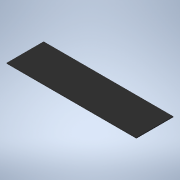
# Autodesk Inventor part: FGR AL-2-PGN-plus-P 160 WKST,PGN-plus-P 160-2-AS-P18Aluminium6.5110452001216049.51650000000000000000
Saved by Autodesk Inventor 2021 (Build 250183000, 183)
## iProperties
Created: 2025-07-30
Part Number: FGR AL-2-PGN-plus-P 160 WKST,PGN-plus-P 160-2-AS-P18Aluminium6.5110452001216049.51650000000000000000
Material: Generic
Catalog Web Link: www.cadenas.de
Description: FGR-Customizable gripper fingers
Vendor: SCHUNK
Document SubType Name: Modeling
Designer: psAdmin
Manufacturer: SCHUNK
Mass: 7.755 g
Surface Area: 159.34 cm^2
Volume: 7.755 cm^3
Density: 1 g/cm^3
Appearance: PSOLRGB-175-175-175
Category: PARTsolutions
Company: SCHUNK
Title: FGR AL-2-PGN-plus-P 160, 110452002
Author: Cadenas PARTsolutions
Comments: Customizable gripper fingers
PSOL_IDENT_0: {$CADENAS_DATA/23d-libs/schunk/greifsysteme/konfigurationen/system_baukasten/easy_finger/easy_finger
PSOL_IDENT_1: _ring.prj},476 {VTYP=3D},{NB=FGR AL-2-PGN-plus-P 160 WKST,PGN-plus-P 160-2-AS-P18Aluminium6.51104520
PSOL_IDENT_2: 01216049.51650000000000000000},{LINA=FGR AL-2-PGN-plus-P 160, 110452002},{NN=FGR},{DATE=13.11.2024 0
PSOL_IDENT_3: 9:26:27},{GEOMDATE=20.06.2024 14:58:27},{VERSION=},{LINEID=10},{WBVAR=BR,BGVR,ASIS,SPANNKONT,CNSMAT,
PSOL_IDENT_4: HUB,RH,X,Y,Z,ABK,DWS,GFL,GFT,PP,PW,RA,EFO,FASE1,FL1,FASE2,FL2,FASE3,FW3,FL3,FASE4,FW4,FL4,WAERMEBE,B
PSOL_IDENT_5: M},{WBNUMERIC=HUB,RH,X,Y,Z,ABK,DWS,GFL,GFT,PP,PW,RA,EFO,FL1,FL2,FASE3,FW3,FL3,FW4,FL4,BM}  {NB=FGR A
PSOL_IDENT_6: L-2-PGN-plus-P 160 WKST,PGN-plus-P 160-2-AS-P18Aluminium6.5110452001216049.51650000000000000000},{LI
PSOL_IDENT_7: NA=FGR AL-2-PGN-plus-P 160, 110452002},{KT=DUMMY},{START=Geometriemodell 2},{VERSION=1},{VER=V1},{MA
PSOL_IDENT_8: TN=3786171200_fgr_gl_ia_v1},{XMLMATN=material|},{XMLMAT=AlZn55MgCu_EN-AW-7075_34365},{TYP=FGR AL-2-P
PSOL_IDENT_9: GN-plus-P 160},{TYPX=PGN-plus-P 160},{TYPXX=PGN-plus-P 160},{TYPXMAT=AL},{BR=PGN-plus-P},{BG=160.0},
PSOL_IDENT_10: {BGVR=PGN-plus-P 160-2-AS-P},{BGVRX='PGN-plus-P 40','PGN-plus-P 40','PGN-plus-P 40-SD','PGN-plus-P 4
PSOL_IDENT_11: 0-SD','PGN-plus-P 40-K','PGN-plus-P 40-K','PGN-plus-P 40-V','PGN-plus-P 40-V','PGN-plus-P 40-P','PGN
PSOL_IDENT_12: -plus-P 40-P','PGN-plus-P 40-AS','PGN-plus-P 40-AS','PGN-plus-P 40-AS-SD','PGN-plus-P 40-AS-SD','PGN
PSOL_IDENT_13: -plus-P 40-AS-K','PGN-plus-P 40-AS-K','PGN-plus-P 40-AS-V','PGN-plus-P 40-AS-V','PGN-plus-P 40-AS-P'
PSOL_IDENT_14: ,'PGN-plus-P 40-AS-P','PGN-plus-P 40-IS','PGN-plus-P 40-IS','PGN-plus-P 40-IS-SD','PGN-plus-P 40-IS-
PSOL_IDENT_15: SD','PGN-plus-P 40-IS-K','PGN-plus-P 40-IS-K','PGN-plus-P 40-IS-V','PGN-plus-P 40-IS-V','PGN-plus-P
PSOL_IDENT_16: 50-1','PGN-plus-P 50-1','PGN-plus-P 50-1-SD','PGN-plus-P 50-1-SD','PGN-plus-P 50-1-K','PGN-plus-P 50
PSOL_IDENT_17: -1-K','PGN-plus-P 50-1-V','PGN-plus-P 50-1-V','PGN-plus-P 50-1-P','PGN-plus-P 50-1-P','PGN-plus-P 50
PSOL_IDENT_18: -2','PGN-plus-P 50-2','PGN-plus-P 50-2-SD','PGN-plus-P 50-2-SD','PGN-plus-P 50-2-K','PGN-plus-P 50-2
PSOL_IDENT_19: -K','PGN-plus-P 50-2-V','PGN-plus-P 50-2-V','PGN-plus-P 50-2-P','PGN-plus-P 50-2-P','PGN-plus-P 50-1
PSOL_IDENT_20: -AS','PGN-plus-P 50-1-AS','PGN-plus-P 50-1-AS-SD','PGN-plus-P 50-1-AS-SD','PGN-plus-P 50-1-AS-K','PG
PSOL_IDENT_21: N-plus-P 50-1-AS-K','PGN-plus-P 50-1-AS-V','PGN-plus-P 50-1-AS-V','PGN-plus-P 50-1-AS-P','PGN-plus-P
PSOL_IDENT_22: 50-1-AS-P','PGN-plus-P 50-2-AS','PGN-plus-P 50-2-AS','PGN-plus-P 50-2-AS-SD','PGN-plus-P 50-2-AS-SD'
PSOL_IDENT_23: ,'PGN-plus-P 50-2-AS-K','PGN-plus-P 50-2-AS-K','PGN-plus-P 50-2-AS-V','PGN-plus-P 50-2-AS-V','PGN-pl
PSOL_IDENT_24: us-P 50-2-AS-P','PGN-plus-P 50-2-AS-P','PGN-plus-P 50-1-IS','PGN-plus-P 50-1-IS','PGN-plus-P 50-1-IS
PSOL_IDENT_25: -SD','PGN-plus-P 50-1-IS-SD','PGN-plus-P 50-1-IS-K','PGN-plus-P 50-1-IS-K','PGN-plus-P 50-1-IS-V','P
PSOL_IDENT_26: GN-plus-P 50-1-IS-V','PGN-plus-P 50-2-IS','PGN-plus-P 50-2-IS','PGN-plus-P 50-2-IS-SD','PGN-plus-P 5
PSOL_IDENT_27: 0-2-IS-SD','PGN-plus-P 50-2-IS-K','PGN-plus-P 50-2-IS-K','PGN-plus-P 50-2-IS-V','PGN-plus-P 50-2-IS-
PSOL_IDENT_28: V','PGN-plus-P 64-1','PGN-plus-P 64-1','PGN-plus-P 64-1-SD','PGN-plus-P 64-1-SD','PGN-plus-P 64-1-K'
PSOL_IDENT_29: ,'PGN-plus-P 64-1-K','PGN-plus-P 64-1-V','PGN-plus-P 64-1-V','PGN-plus-P 64-1-P','PGN-plus-P 64-1-P'
PSOL_IDENT_30: ,'PGN-plus-P 64-2','PGN-plus-P 64-2','PGN-plus-P 64-2-SD','PGN-plus-P 64-2-SD','PGN-plus-P 64-2-K','
PSOL_IDENT_31: PGN-plus-P 64-2-K','PGN-plus-P 64-2-V','PGN-plus-P 64-2-V','PGN-plus-P 64-2-P','PGN-plus-P 64-2-P','
PSOL_IDENT_32: PGN-plus-P 64-1-AS','PGN-plus-P 64-1-AS','PGN-plus-P 64-1-AS-SD','PGN-plus-P 64-1-AS-SD','PGN-plus-P
PSOL_IDENT_33: 64-1-AS-K','PGN-plus-P 64-1-AS-K','PGN-plus-P 64-1-AS-V','PGN-plus-P 64-1-AS-V','PGN-plus-P 64-1-AS
PSOL_IDENT_34: -P','PGN-plus-P 64-1-AS-P','PGN-plus-P 64-2-AS','PGN-plus-P 64-2-AS','PGN-plus-P 64-1-IS','PGN-plus-
PSOL_IDENT_35: P 64-1-IS','PGN-plus-P 64-1-IS-SD','PGN-plus-P 64-1-IS-SD','PGN-plus-P 64-1-IS-K','PGN-plus-P 64-1-I
PSOL_IDENT_36: S-K','PGN-plus-P 64-1-IS-V','PGN-plus-P 64-1-IS-V','PGN-plus-P 64-2-IS','PGN-plus-P 64-2-IS','PGN-pl
PSOL_IDENT_37: us-P 64-2-IS-SD','PGN-plus-P 64-2-IS-SD','PGN-plus-P 64-2-IS-K','PGN-plus-P 64-2-IS-K','PGN-plus-P 6
PSOL_IDENT_38: 4-2-V','PGN-plus-P 64-2-V','PGN-plus-P 80-1','PGN-plus-P 80-1','PGN-plus-P 80-1-SD','PGN-plus-P 80-1
PSOL_IDENT_39: -SD','PGN-plus-P 80-1-K','PGN-plus-P 80-1-K','PGN-plus-P 80-1-V','PGN-plus-P 80-1-V','PGN-plus-P 80-
PSOL_IDENT_40: 1-P','PGN-plus-P 80-1-P','PGN-plus-P 80-2','PGN-plus-P 80-2','PGN-plus-P 80-2-SD','PGN-plus-P 80-2-S
PSOL_IDENT_41: D','PGN-plus-P 80-2-K','PGN-plus-P 80-2-K','PGN-plus-P 80-2-V','PGN-plus-P 80-2-V','PGN-plus-P 80-2-
PSOL_IDENT_42: P','PGN-plus-P 80-2-P','PGN-plus-P 80-1-AS','PGN-plus-P 80-1-AS','PGN-plus-P 80-1-AS-SD','PGN-plus-P
PSOL_IDENT_43: 80-1-AS-SD','PGN-plus-P 80-1-AS-K','PGN-plus-P 80-1-AS-K','PGN-plus-P 80-1-AS-V','PGN-plus-P 80-1-A
PSOL_IDENT_44: S-V','PGN-plus-P 80-1-AS-P','PGN-plus-P 80-1-AS-P','PGN-plus-P 80-2-AS','PGN-plus-P 80-2-AS','PGN-pl
PSOL_IDENT_45: us-P 80-2-AS-SD', 'PGN-plus-P 80-2-AS-SD','PGN-plus-P 80-2-AS-K','PGN-plus-P 80-2-AS-K','PGN-plus-P
PSOL_IDENT_46: 80-2-AS-V','PGN-plus-P 80-2-AS-V','PGN-plus-P 80-2-AS-P','PGN-plus-P 80-2-AS-P','PGN-plus-P 80-1-IS'
PSOL_IDENT_47: ,'PGN-plus-P 80-1-IS','PGN-plus-P 80-1-IS-SD','PGN-plus-P 80-1-IS-SD','PGN-plus-P 80-1-IS-K','PGN-pl
PSOL_IDENT_48: us-P 80-1-IS-K','PGN-plus-P 80-1-IS-V','PGN-plus-P 80-1-IS-V','PGN-plus-P 80-2-IS','PGN-plus-P 80-2-
PSOL_IDENT_49: IS','PGN-plus-P 80-2-IS-SD','PGN-plus-P 80-2-IS-SD','PGN-plus-P 80-2-IS-K','PGN-plus-P 80-2-IS-K','P
PSOL_IDENT_50: GN-plus-P 80-2-IS-V','PGN-plus-P 80-2-IS-V','PGN-plus-P 100-1','PGN-plus-P 100-1','PGN-plus-P 100-1-
PSOL_IDENT_51: SD','PGN-plus-P 100-1-SD','PGN-plus-P 100-1-K','PGN-plus-P 100-1-K','PGN-plus-P 100-1-V','PGN-plus-P
PSOL_IDENT_52: 100-1-V','PGN-plus-P 100-1-P','PGN-plus-P 100-1-P','PGN-plus-P 100-2','PGN-plus-P 100-2','PGN-plus-
PSOL_IDENT_53: P 100-2-SD','PGN-plus-P 100-2-SD','PGN-plus-P 100-2-K','PGN-plus-P 100-2-K','PGN-plus-P 100-2-V','PG
PSOL_IDENT_54: N-plus-P 100-2-V','PGN-plus-P 100-2-P','PGN-plus-P 100-2-P','PGN-plus-P 100-1-AS','PGN-plus-P 100-1-
PSOL_IDENT_55: AS','PGN-plus-P 100-1-AS-SD','PGN-plus-P 100-1-AS-SD','PGN-plus-P 100-1-AS-K','PGN-plus-P 100-1-AS-K'
PSOL_IDENT_56: ,'PGN-plus-P 100-1-AS-V','PGN-plus-P 100-1-AS-V','PGN-plus-P 100-1-AS-P','PGN-plus-P 100-1-AS-P','PG
PSOL_IDENT_57: N-plus-P 100-2-AS','PGN-plus-P 100-2-AS','PGN-plus-P 100-2-AS-SD','PGN-plus-P 100-2-AS-SD','PGN-plus
PSOL_IDENT_58: -P 100-2-AS-K','PGN-plus-P 100-2-AS-K','PGN-plus-P 100-2-AS-V','PGN-plus-P 100-2-AS-V','PGN-plus-P 1
PSOL_IDENT_59: 00-2-AS-P','PGN-plus-P 100-2-AS-P','PGN-plus-P 100-1-IS','PGN-plus-P 100-1-IS','PGN-plus-P 100-1-IS-
PSOL_IDENT_60: SD','PGN-plus-P 100-1-IS-SD','PGN-plus-P 100-1-IS-K','PGN-plus-P 100-1-IS-K','PGN-plus-P 100-1-IS-V'
PSOL_IDENT_61: ,'PGN-plus-P 100-1-IS-V','PGN-plus-P 100-2-IS','PGN-plus-P 100-2-IS','PGN-plus-P 100-2-IS-SD','PGN-p
PSOL_IDENT_62: lus-P 100-2-IS-SD','PGN-plus-P 100-2-IS-K','PGN-plus-P 100-2-IS-K','PGN-plus-P 100-2-IS-V','PGN-plus
PSOL_IDENT_63: -P 100-2-IS-V','PGN-plus-P 125-1','PGN-plus-P 125-1','PGN-plus-P 125-1-SD','PGN-plus-P 125-1-SD','PG
PSOL_IDENT_64: N-plus-P 125-1-K','PGN-plus-P 125-1-K','PGN-plus-P 125-1-V','PGN-plus-P 125-1-V','PGN-plus-P 125-1-P'
PSOL_IDENT_65: ,'PGN-plus-P 125-1-P','PGN-plus-P 125-2','PGN-plus-P 125-2','PGN-plus-P 125-2-SD','PGN-plus-P 125-2-
PSOL_IDENT_66: SD','PGN-plus-P 125-2-K','PGN-plus-P 125-2-K','PGN-plus-P 125-2-V','PGN-plus-P 125-2-V','PGN-plus-P
PSOL_IDENT_67: 125-2-P','PGN-plus-P 125-2-P','PGN-plus-P 125-1-AS','PGN-plus-P 125-1-AS','PGN-plus-P 125-1-AS-SD','
PSOL_IDENT_68: PGN-plus-P 125-1-AS-SD','PGN-plus-P 125-1-AS-K','PGN-plus-P 125-1-AS-K','PGN-plus-P 125-1-AS-V','PGN
PSOL_IDENT_69: -plus-P 125-1-AS-V','PGN-plus-P 125-1-AS-P','PGN-plus-P 125-1-AS-P','PGN-plus-P 125-2-AS','PGN-plus-
PSOL_IDENT_70: P 125-2-AS','PGN-plus-P 125-2-AS-SD','PGN-plus-P 125-2-AS-SD','PGN-plus-P 125-2-AS-K','PGN-plus-P 12
PSOL_IDENT_71: 5-2-AS-K','PGN-plus-P 125-2-AS-V','PGN-plus-P 125-2-AS-V','PGN-plus-P 125-2-AS-P','PGN-plus-P 125-2-
PSOL_IDENT_72: AS-P','PGN-plus-P 125-1-IS','PGN-plus-P 125-1-IS','PGN-plus-P 125-1-IS-SD','PGN-plus-P 125-1-IS-SD','
PSOL_IDENT_73: PGN-plus-P 125-1-IS-K','PGN-plus-P 125-1-IS-K','PGN-plus-P 125-1-IS-V','PGN-plus-P 125-1-IS-V','PGN-
PSOL_IDENT_74: plus-P 125-2-IS','PGN-plus-P 125-2-IS','PGN-plus-P 125-2-IS-SD','PGN-plus-P 125-2-IS-SD','PGN-plus-P
PSOL_IDENT_75: 125-2-IS-K','PGN-plus-P 125-2-IS-K','PGN-plus-P 125-2-IS-V','PGN-plus-P 125-2-IS-V','PGN-plus-P 160
PSOL_IDENT_76: -1','PGN-plus-P 160-1','PGN-plus-P 160-1-SD','PGN-plus-P 160-1-SD','PGN-plus-P 160-1-K','PGN-plus-P
PSOL_IDENT_77: 160-1-K','PGN-plus-P 160-1-V','PGN-plus-P 160-1-V','PGN-plus-P 160-1-P','PGN-plus-P 160-1-P','PGN-pl
PSOL_IDENT_78: us-P 160-2','PGN-plus-P 160-2','PGN-plus-P 160-2-SD','PGN-plus-P 160-2-SD','PGN-plus-P 160-2-K','PGN
PSOL_IDENT_79: -plus-P 160-2-K','PGN-plus-P 160-2-V','PGN-plus-P 160-2-V','PGN-plus-P 160-2-P','PGN-plus-P 160-2-P'
PSOL_IDENT_80: ,'PGN-plus-P 160-1-AS','PGN-plus-P 160-1-AS','PGN-plus-P 160-1-AS-SD','PGN-plus-P 160-1-AS-SD','PGN-
PSOL_IDENT_81: plus-P 160-1-AS-K','PGN-plus-P 160-1-AS-K','PGN-plus-P 160-1-AS-V','PGN-plus-P 160-1-AS-V','PGN-plus
PSOL_IDENT_82: -P 160-1-AS-P','PGN-plus-P 160-1-AS-P','PGN-plus-P 160-2-AS','PGN-plus-P 160-2-AS','PGN-plus-P 160-2
PSOL_IDENT_83: -AS-SD','PGN-plus-P 160-2-AS-SD','PGN-plus-P 160-2-AS-K','PGN-plus-P 160-2-AS-K','PGN-plus-P 160-2-A
PSOL_IDENT_84: S-V','PGN-plus-P 160-2-AS-V','PGN-plus-P 160-2-AS-P','PGN-plus-P 160-2-AS-P','PGN-plus-P 160-1-IS','
PSOL_IDENT_85: PGN-plus-P 160-1-IS','PGN-plus-P 160-1-IS-SD','PGN-plus-P 160-1-IS-SD','PGN-plus-P 160-1-IS-K','PGN-
PSOL_IDENT_86: plus-P 160-1-IS-K','PGN-plus-P 160-1-IS-V','PGN-plus-P 160-1-IS-V','PGN-plus-P 160-2-IS','PGN-plus-P
PSOL_IDENT_87: 160-2-IS','PGN-plus-P 160-2-IS-SD','PGN-plus-P 160-2-IS-SD','PGN-plus-P 160-2-IS-K','PGN-plus-P 160
PSOL_IDENT_88: -2-IS-K','PGN-plus-P 160-2-IS-V','PGN-plus-P 160-2-IS-V','PGN-plus-P 200-1','PGN-plus-P 200-1','PGN-
PSOL_IDENT_89: plus-P 200-1-SD','PGN-plus-P 200-1-SD','PGN-plus-P 200-1-K','PGN-plus-P 200-1-K','PGN-plus-P 200-1-V'
PSOL_IDENT_90: ,'PGN-plus-P 200-1-V','PGN-plus-P 200-1-P','PGN-plus-P 200-1-P','PGN-plus-P 200-2','PGN-plus-P 200-2'
PSOL_IDENT_91: ,'PGN-plus-P 200-2-SD','PGN-plus-P 200-2-SD','PGN-plus-P 200-2-K','PGN-plus-P 200-2-K','PGN-plus-P 2
PSOL_IDENT_92: 00-2-V','PGN-plus-P 200-2-V','PGN-plus-P 200-2-P','PGN-plus-P 200-2-P','PGN-plus-P 200-1-AS','PGN-pl
PSOL_IDENT_93: us-P 200-1-AS','PGN-plus-P 200-1-AS-SD','PGN-plus-P 200-1-AS-SD','PGN-plus-P 200-1-AS-K','PGN-plus-P
PSOL_IDENT_94: 200-1-AS-K','PGN-plus-P 200-1-AS-V','PGN-plus-P 200-1-AS-V','PGN-plus-P 200-1-AS-P','PGN-plus-P 200
PSOL_IDENT_95: -1-AS-P','PGN-plus-P 200-2-AS','PGN-plus-P 200-2-AS','PGN-plus-P 200-2-AS-SD','PGN-plus-P 200-2-AS-S
PSOL_IDENT_96: D','PGN-plus-P 200-2-AS-K','PGN-plus-P 200-2-AS-K','PGN-plus-P 200-2-AS-V','PGN-plus-P 200-2-AS-V','
PSOL_IDENT_97: PGN-plus-P 200-2-AS-P','PGN-plus-P 200-2-AS-P','PGN-plus-P 200-1-IS','PGN-plus-P 200-1-IS','PGN-plus
PSOL_IDENT_98: -P 200-1-IS-SD','PGN-plus-P 200-1-IS-SD','PGN-plus-P 200-1-IS-K','PGN-plus-P 200-1-IS-K','PGN-plus-P
PSOL_IDENT_99: 200-1-IS-V','PGN-plus-P 200-1-IS-V','PGN-plus-P 200-2-IS','PGN-plus-P 200-2-IS','PGN-plus-P 200-2-I
PSOL_IDENT_100: S-SD','PGN-plus-P 200-2-IS-SD','PGN-plus-P 200-2-IS-K','PGN-plus-P 200-2-IS-K','PGN-plus-P 200-2-IS-
PSOL_IDENT_101: V','PGN-plus-P 200-2-IS-V','PGN-plus-P 240-1','PGN-plus-P 240-1','PGN-plus-P 240-1-SD','PGN-plus-P 2
PSOL_IDENT_102: 40-1-SD','PGN-plus-P 240-1-K','PGN-plus-P 240-1-K','PGN-plus-P 240-1-V','PGN-plus-P 240-1-V','PGN-pl
PSOL_IDENT_103: us-P 240-1-P','PGN-plus-P 240-1-P','PGN-plus-P 240-2','PGN-plus-P 240-2','PGN-plus-P 240-2-SD','PGN-
PSOL_IDENT_104: plus-P 240-2-SD','PGN-plus-P 240-2-K','PGN-plus-P 240-2-K','PGN-plus-P 240-2-V','PGN-plus-P 240-2-V'
PSOL_IDENT_105: ,'PGN-plus-P 240-2-P','PGN-plus-P 240-2-P', 'PGN-plus-P 240-1-AS','PGN-plus-P 240-1-AS','PGN-plus-P
PSOL_IDENT_106: 240-1-AS-SD','PGN-plus-P 240-1-AS-SD','PGN-plus-P 240-1-AS-K','PGN-plus-P 240-1-AS-K','PGN-plus-P 24
PSOL_IDENT_107: 0-1-AS-V','PGN-plus-P 240-1-AS-V','PGN-plus-P 240-1-AS-P','PGN-plus-P 240-1-AS-P', 'PGN-plus-P 240-2
PSOL_IDENT_108: -AS','PGN-plus-P 240-2-AS','PGN-plus-P 240-2-AS-SD','PGN-plus-P 240-2-AS-SD','PGN-plus-P 240-2-AS-K'
PSOL_IDENT_109: ,'PGN-plus-P 240-2-AS-K','PGN-plus-P 240-2-AS-V','PGN-plus-P 240-2-AS-V','PGN-plus-P 240-2-AS-P','PG
PSOL_IDENT_110: N-plus-P 240-2-AS-P', 'PGN-plus-P 240-1-IS','PGN-plus-P 240-1-IS','PGN-plus-P 240-1-IS-SD','PGN-plus
PSOL_IDENT_111: -P 240-1-IS-SD','PGN-plus-P 240-1-IS-K','PGN-plus-P 240-1-IS-K','PGN-plus-P 240-1-IS-V','PGN-plus-P
PSOL_IDENT_112: 240-1-IS-V', 'PGN-plus-P 240-2-IS','PGN-plus-P 240-2-IS','PGN-plus-P 240-2-IS-SD','PGN-plus-P 240-2-
PSOL_IDENT_113: IS-SD','PGN-plus-P 240-2-IS-K','PGN-plus-P 240-2-IS-K','PGN-plus-P 240-2-IS-V','PGN-plus-P 240-2-IS-
PSOL_IDENT_114: V','PGN-plus-P 300-1','PGN-plus-P 300-1','PGN-plus-P 300-1-SD','PGN-plus-P 300-1-SD','PGN-plus-P 300
PSOL_IDENT_115: -1-K','PGN-plus-P 300-1-K','PGN-plus-P 300-1-V','PGN-plus-P 300-1-V','PGN-plus-P 300-1-P','PGN-plus-
PSOL_IDENT_116: P 300-1-P','PGN-plus-P 300-2','PGN-plus-P 300-2','PGN-plus-P 300-2-SD','PGN-plus-P 300-2-SD','PGN-pl
PSOL_IDENT_117: us-P 300-2-K','PGN-plus-P 300-2-K','PGN-plus-P 300-2-V','PGN-plus-P 300-2-V','PGN-plus-P 300-2-P','P
PSOL_IDENT_118: GN-plus-P 300-2-P', 'PGN-plus-P 300-1-AS','PGN-plus-P 300-1-AS','PGN-plus-P 300-1-AS-SD','PGN-plus-P
PSOL_IDENT_119: 300-1-AS-SD','PGN-plus-P 300-1-AS-K','PGN-plus-P 300-1-AS-K','PGN-plus-P 300-1-AS-V','PGN-plus-P 30
PSOL_IDENT_120: 0-1-AS-V','PGN-plus-P 300-1-AS-P','PGN-plus-P 300-1-AS-P', 'PGN-plus-P 300-2-AS','PGN-plus-P 300-2-A
PSOL_IDENT_121: S','PGN-plus-P 300-2-AS-SD','PGN-plus-P 300-2-AS-SD','PGN-plus-P 300-2-AS-K','PGN-plus-P 300-2-AS-K'
PSOL_IDENT_122: ,'PGN-plus-P 300-2-AS-V','PGN-plus-P 300-2-AS-V','PGN-plus-P 300-2-AS-P','PGN-plus-P 300-2-AS-P', 'P
PSOL_IDENT_123: GN-plus-P 300-1-IS','PGN-plus-P 300-1-IS','PGN-plus-P 300-1-IS-SD','PGN-plus-P 300-1-IS-SD','PGN-plu
PSOL_IDENT_124: s-P 300-1-IS-K','PGN-plus-P 300-1-IS-K','PGN-plus-P 300-1-IS-V','PGN-plus-P 300-1-IS-V', 'PGN-plus-P
PSOL_IDENT_125: 300-2-IS','PGN-plus-P 300-2-IS','PGN-plus-P 300-2-IS-SD','PGN-plus-P 300-2-IS-SD','PGN-plus-P 300-2
PSOL_IDENT_126: -IS-K','PGN-plus-P 300-2-IS-K','PGN-plus-P 300-2-IS-V','PGN-plus-P 300-2-IS-V','PGN-plus-P 380-1','P
PSOL_IDENT_127: GN-plus-P 380-1','PGN-plus-P 380-1-SD','PGN-plus-P 380-1-SD','PGN-plus-P 380-1-K','PGN-plus-P 380-1-
PSOL_IDENT_128: K','PGN-plus-P 380-1-V','PGN-plus-P 380-1-V','PGN-plus-P 380-1-P','PGN-plus-P 380-1-P','PGN-plus-P 3
PSOL_IDENT_129: 80-2','PGN-plus-P 380-2','PGN-plus-P 380-2-SD','PGN-plus-P 380-2-SD','PGN-plus-P 380-2-K','PGN-plus-
PSOL_IDENT_130: P 380-2-K','PGN-plus-P 380-2-V','PGN-plus-P 380-2-V','PGN-plus-P 380-2-P','PGN-plus-P 380-2-P', 'PGN
PSOL_IDENT_131: -plus-P 380-1-AS','PGN-plus-P 380-1-AS','PGN-plus-P 380-1-AS-SD','PGN-plus-P 380-1-AS-SD','PGN-plus-
PSOL_IDENT_132: P 380-1-AS-K','PGN-plus-P 380-1-AS-K','PGN-plus-P 380-1-AS-V','PGN-plus-P 380-1-AS-V','PGN-plus-P 38
PSOL_IDENT_133: 0-1-AS-P','PGN-plus-P 380-1-AS-P', 'PGN-plus-P 380-2-AS','PGN-plus-P 380-2-AS','PGN-plus-P 380-2-AS-
PSOL_IDENT_134: SD','PGN-plus-P 380-2-AS-SD','PGN-plus-P 380-2-AS-K','PGN-plus-P 380-2-AS-K','PGN-plus-P 380-2-AS-V'
PSOL_IDENT_135: ,'PGN-plus-P 380-2-AS-V','PGN-plus-P 380-2-AS-P','PGN-plus-P 380-2-AS-P', 'PGN-plus-P 380-1-IS','PGN
PSOL_IDENT_136: -plus-P 380-1-IS','PGN-plus-P 380-1-IS-SD','PGN-plus-P 380-1-IS-SD','PGN-plus-P 380-1-IS-K','PGN-plu
PSOL_IDENT_137: s-P 380-1-IS-K','PGN-plus-P 380-1-IS-V','PGN-plus-P 380-1-IS-V', 'PGN-plus-P 380-2-IS','PGN-plus-P 3
PSOL_IDENT_138: 80-2-IS','PGN-plus-P 380-2-IS-SD','PGN-plus-P 380-2-IS-SD','PGN-plus-P 380-2-IS-K','PGN-plus-P 380-2
PSOL_IDENT_139: -IS-K','PGN-plus-P 380-2-IS-V','PGN-plus-P 380-2-IS-V'},{BGVRZ=116.800},{BGVRXX=77.0},{ZBAX=109.0},{
PSOL_IDENT_140: IDNR=1317660},{ASIS=1},{ASISX=<'1','Außengreifen','aussengreifen.png'>,'2','Innnengreifen','innengre
PSOL_IDENT_141: ifen.png'},{ASISXX=AS},{SPANNKONT=2},{SPANNKONTX='1', 'Gerader Greiferfinger', 'startmodell_1.png', '
PSOL_IDENT_142: 2' , 'Greiferfinger mit nach innen abgesetzter Greiffläche', 'startmodell_2.png', '3' , 'Greiferfing
PSOL_IDENT_143: er mit nach außen abgesetzter Greiffläche', 'startmodell_3.png', '4' , 'Greiferfinger mit nach innen
PSOL_IDENT_144: abgesetzter und abgerundeter Greiffläche', 'startmodell_4.png', '5' , 'Greiferfinger mit nach außen
PSOL_IDENT_145: abgesetzter und abgerundeter Greiffläche', 'startmodell_5.png', '6' , 'Greiferfinger mit nach innen
PSOL_IDENT_146: abgesetzter Greiffläche und vertikalem Prisma', 'startmodell_6.png','8' , 'Greiferfinger mit horizo
PSOL_IDENT_147: ntalem Prisma', 'startmodell_8.png'},{CNSMAT=Aluminium},{HUB=8.0},{HMAX=8.0},{RH=6.5},{HMAXX=8.0},{R
PSOL_IDENT_148: HB=2.0},{GFM=38.50},{GFMAS=38.50},{GFMIS=70.50},{X=110.0},{XMIN=56.0},{XMAX=113.0},{XTEST=[56:113/0.
PSOL_IDENT_149: 1]},{MAXX=113.0},{Y=45.0},{YMIN=27.0},{YMAX=60.0},{MAXY=60.0},{Z=200.0},{ZMIN=32.0},{ZMAX=200.0},{ZM
PSOL_IDENT_150: AXX=100.0},{MAXZ=200.0},{ABK=12.00},{ABKMIN=12.00},{ABKMAX=37.50},{DWS=165.0},{DWSX=[68:222]},{DWSMI
PSOL_IDENT_151: N=68.000},{DWSMAX=222.000},{DWSMAXX=111.0},{DWSXX=1.000},{DWSZ=1.000},{DWS1V=70.0},{DWS1H=110.0},{DW
PSOL_IDENT_152: S2V=134.0},{GWI=1.0},{GFL=160.0},{GFLX=[1:169.4]},{GFLMIN=1.00},{GFLMAX=169.40},{GFT=49.50},{GFTX=[4
PSOL_IDENT_153: 9.5:49.5/0.1]},{GFTMIN=49.50},{GFTMINTH=-217577236067824.12},{GFTMAX=49.50},{GFT1V=2.00},{GFT1H=22.0
PSOL_IDENT_154: 0},{GFT2V=34.00},{GFT2H=54.00},{SKS=10.6},{PP=0.0},{PPX=[0]},{PPMIN=0.0},{PPMAX=0.0},{PUK=0.00},{PUK
PSOL_IDENT_155: Z=88.50},{PUKX=0.00},{PW=0.0},{PWX=[0]},{PWMIN=120},{PWMAX=120},{PWTH=120.0},{PWTHX=180.000},{ALPHA=
PSOL_IDENT_156: 0.000},{RA=0.0},{RAX=[0]},{RAMIN=1.0},{RAMAX=44},{EFO=0.0},{EFOX=[0]},{EFOMAX=0.10},{FASE1=0},{FASE1
PSOL_IDENT_157: X='0','ohne Fase 1','kein_bild.png','1','mit Fase 1','fase_1.png'},{FW1=0.0},{FL1=0.0},{FL1MIN=0.0},
PSOL_IDENT_158: {FL1MAX=0.0},{FASE2=0},{FASE2X='0','ohne Fase 2','kein_bild.png','1','mit Fase 2','fase_2.png'},{FW2=
PSOL_IDENT_159: 0.0},{FL2=0.0},{FL2MIN=0.0},{FL2MAX=0.0},{FASE3=0},{FW3=0.0},{FW3MIN=0.0},{FW3MAX=0.0},{FL3=0.0},{FL
PSOL_IDENT_160: 3MIN=0.0},{FL3MAX=0.00},{FASE4=0},{FASE4X='0','ohne Fase 4','kein_bild.png','1','mit Fase 4','fase_4
PSOL_IDENT_161: _glatt.png'},{FW4=0.0},{FW4MIN=0.0},{FW4MAX=0.0},{FL4=0.0},{FL4MIN=0.0},{FL4MAX=0.00},{ROH=1.457},{Z
PSOL_IDENT_162: ULFM=3.800},{VALFM=true},{VOL=537767.200},{VFASE1=0.00},{VFASE2=0.00},{VFASE3=0.00},{VFASE4=0.00},{G
PSOL_IDENT_163: FTXX=2.00},{STX1=20.00},{STX2=20.00},{EST=17.0},{AB=32.0},{ZD=14.0},{ZT=4.0},{DB=11.0},{SD=18.0},{ST=
PSOL_IDENT_164: 20.00},{RI=8.2},{L=6.500},{LX=-31.000},{L1=1.000},{L1X=-0.000},{L2=1.000},{LA=82.500},{GANS=M10},{PB
PSOL_IDENT_165: O=11.0},{DPB=11.00},{RPO=3},{AQB=2.8},{SCHT=0.75},{SCHL=17.40},{SCHH=6.40},{SCHP=5.00},{TYPALU=3.00}
PSOL_IDENT_166: ,{SCHGD=10.0},{SCHGL=35.0},{LZ=5 Werktage},{SAPLZ=5},{VK=272.00},{VKB=226.11},{VKZ=33.92},{VKX=11.31
PSOL_IDENT_167: },{VKP=0.00},{VKW=0.00},{ZX=200.0},{ZXX=100.0},{XX=113.0},{XXX=56.5},{SPERR=0.00},{WC=3786171200_fgr
PSOL_IDENT_168: _gl_ia_v1.prt},{MN=3786171200_FGR_GL_IA_V1},{XMLX=dim|15},{XMLY=dim|14},{XMLZ=dim|13},{XMLAB=dim|35}
PSOL_IDENT_169: ,{XMLABK=dim|71},{XMLFL1=dim|188},{XMLFL2=dim|151},{XMLFL3=dim|272},{XMLFW3=dim|274},{XMLFL4=dim|212
PSOL_IDENT_170: },{XMLFW4=dim|211},{XMLGFL=dim|70},{XMLGFT=dim|68},{XMLRA=},{XMLRI=},{XMLPW=},{XMLDWS=para|DWS},{XML
PSOL_IDENT_171: GFM=para|GFM},{XMLRH=},{XMLEFO=},{XMLPP=},{XMLASIS=para|ASIS},{XMLVER=para|1|VER},{ANZ=2},{SG3D=8.0}
PSOL_IDENT_172: ,{WAERMEBEX='',''},{WAERMEBE=},{SAPWAERMEBE=10},{DICHTE=2.71},{BM=2}
NB: FGR AL-2-PGN-plus-P 160 WKST,PGN-plus-P 160-2-AS-P18Aluminium6.5110452001216049.51650000000000000000
NN: FGR
NT: Customizable gripper fingers
NBSYN: $TYP. WKST,$BGVR.$ASIS.$HUB.$CNSMAT.$RH.$X.$Y.$Z.$ABK.$GFL.$GFT.$DWS.$PP.$PW.$RA.$EFO.$FASE1.$FW1.$FL1.$FASE2.$FW2.$FL2.$FASE3.$FW3.$FL3.$FASE4.$FW4.$FL4.
LINA: FGR AL-2-PGN-plus-P 160, 110452002
CATALOG: SCHUNK
VER: V1
XMLMATN: material|
BR: PGN-plus-P
BGVR: PGN-plus-P 160-2-AS-P
ASIS: O.D. gripping
SPANNKONT: Gripper finger with inwardly stepped gripping surface
CNSMAT: Aluminium AlZnMgCu1,5
HUB: 8
RH: 6.5
X: 110
Y: 45
Z: 200
ABK: 12
DWS: 165
GFL: 160
GFT: 49.5
PP: 0
PW: 0
RA: 0
RAMIN: 1
EFO: 0
FASE1: without chamfer 1
FL1: 0
FASE2: without chamfer 2
FL2: 0
FASE3: without chamfer 3
FW3: 0
FL3: 0
FASE4: without chamfer 4
FW4: 0
FL4: 0
XMLX: dim|15
XMLY: dim|14
XMLZ: dim|13
XMLAB: dim|35
XMLDWS: para|DWS
XMLGFM: para|GFM
XMLASIS: para|ASIS
XMLVER: para|1|VER
BM: 2
SUPPLIER: SCHUNK
ARTICLENO: FGR AL-2-PGN-plus-P 160 WKST,PGN-plus-P 160-2-AS-P18Aluminium6.5110452001216049.51650000000000000000
BOMINFO: FGR AL-2-PGN-plus-P 160, 110452002
CREATOR: CADENAS GmbH
Autodesk Inventor part; units mm, degrees
sketch "Sketch_3" plane through (0, 0, 0) normal (0, 1, 0) x (-1, 0, 0)
  line L0 (82.5, -23.5) -> (82.5, 23.5)
  line L1 (82.5, 23.5) -> (-82.5, 23.5)
  line L2 (-82.5, 23.5) -> (-82.5, -23.5)
  line L3 (-82.5, -23.5) -> (82.5, -23.5)
  constraints: 8 end point
extrude "Extrusion1" add sketch "Sketch_3" along normal blind 1
ref_plane "IP_WKST_XY" through (0, 0, 0) normal (0, 1, 0) x (1, 0, 0)
ref_plane "IP_WKST_YZ" through (0, 0, 0) normal (1, 0, 0) x (0, 0, -1)
ref_plane "IP_WKST_ZX" through (0, 0, 0) normal (0, 0, -1) x (0, 1, 0)
body "Solid1"
